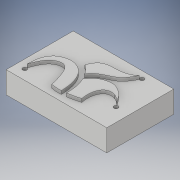
# Autodesk Inventor part: cimproj
Saved by Autodesk Inventor 2019 (Build 230136000, 136)
## iProperties
Created: 2021-02-26
Part Number: cimproj
Material: Generic
Document SubType Name: Modeling
Designer: Davron
Density: 1 g/cm^3
Appearance: Default
Author: Davron
Autodesk Inventor part; units mm, degrees
ref_plane "YZ Plane" through (0, 0, 0) normal (1, 0, 0) x (0, 1, 0)
ref_plane "XZ Plane" through (0, 0, 0) normal (0, 1, 0) x (-1, 0, 0)
ref_plane "XY Plane" through (0, 0, 0) normal (0, 0, 1) x (1, 0, 0)
sketch "Sketch1" plane through (0, 0, 0) normal (0, 1, 0) x (-1, 0, 0)
  line L0 (105.8864, -9.1713) -> (29.6864, -9.1713)
  line L1 (29.6864, -9.1713) -> (29.6864, -59.9713)
  line L2 (29.6864, -59.9713) -> (105.8864, -59.9713)
  line L3 (105.8864, -59.9713) -> (105.8864, -9.1713)
  point P0 (0, 0)
  dimension "d0" = 76.2
  dimension "d1" = 50.8
  constraints: 8 end point, 3 perpendicular, 1 horizontal
  measures "d0" distance of L0.start L0.end
  measures "d1" distance of L0.end L1.end
extrude "Extrusion1" add sketch "Sketch1" along normal blind 16.51
sketch "Sketch2" plane through (0, 16.51, 0) normal (0, 1, 0) x (1, 0, 0)
  line L0 (-99.1001, 18.3012) -> (-96.0417, 26.9953) construction
  line L1 (-96.0417, 26.9953) -> (-92.1887, 31.3423) construction
  line L2 (-92.1887, 31.3423) -> (-84.285, 34.3061) construction
  line L3 (-84.285, 34.3061) -> (-80.6296, 29.3664) construction
  line L4 (-80.6296, 29.3664) -> (-77.2705, 18.3012) construction
  line L5 (-77.2705, 18.3012) -> (-76.579, 14.4191) construction
  spline S0 degree 4 poles (-99.1001, 18.3012) (-96.0417, 26.9953) (-92.1887, 31.3423) (-84.285, 34.3061) (-80.6296, 29.3664) (-77.2705, 18.3012) (-76.579, 14.4191) knots 1 1 1 1 1 2 3 4 4 4 4 4
  line L6 (-99.1001, 18.3012) -> (-99.1001, 25.8499) construction
  line L7 (-99.1001, 25.8499) -> (-96.5674, 31.3423) construction
  line L8 (-96.5674, 31.3423) -> (-93.9607, 34.9573) construction
  line L9 (-93.9607, 34.9573) -> (-88.2369, 37.0386) construction
  line L10 (-88.2369, 37.0386) -> (-83.2313, 37.9368) construction
  line L11 (-83.2313, 37.9368) -> (-75.6293, 34.8836) construction
  line L12 (-75.6293, 34.8836) -> (-71.3593, 29.3664) construction
  line L13 (-71.3593, 29.3664) -> (-68.785, 20.2226) construction
  line L14 (-68.785, 20.2226) -> (-68.785, 13.8588) construction
  spline S1 degree 4 poles (-99.1001, 18.3012) (-99.1001, 25.8499) (-96.5674, 31.3423) (-93.9607, 34.9573) (-88.2369, 37.0386) (-83.2313, 37.9368) (-75.6293, 34.8836) (-71.3593, 29.3664) (-68.785, 20.2226) (-68.785, 13.8588) knots 1 1 1 1 1 2 3 4 5 6 7 7 7 7 7
  line L15 (-68.2598, 29.584) -> (-66.503, 25.2471) construction
  line L16 (-66.503, 25.2471) -> (-65.2915, 22.9111) construction
  line L17 (-65.2915, 22.9111) -> (-65.2915, 14.27) construction
  spline S2 degree 3 poles (-68.2598, 29.584) (-66.503, 25.2471) (-65.2915, 22.9111) (-65.2915, 14.27) knots 1 1 1 1 2 2 2 2
  spline S3 degree 2 poles (-70.7555, 33.4961) (-73.1331, 37.1458) (-76.6265, 39.605) knots 0 0 0 1 1 1
  line L18 (-76.6265, 39.605) -> (-71.5951, 54.9343) construction
  line L19 (-71.5951, 54.9343) -> (-60.3667, 43.5663) construction
  line L20 (-60.3667, 43.5663) -> (-49.0964, 53.1455) construction
  spline S4 degree 3 poles (-76.6265, 39.605) (-71.5951, 54.9343) (-60.3667, 43.5663) (-49.0964, 53.1455) knots 1 1 1 1 2 2 2 2
  line L21 (-65.2915, 14.27) -> (-59.8318, 14.9374) construction
  line L22 (-59.8318, 14.9374) -> (-55.9104, 16.3841) construction
  line L23 (-55.9104, 16.3841) -> (-55.7779, 16.3841) construction
  spline S5 degree 3 poles (-65.2915, 14.27) (-59.8318, 14.9374) (-55.9104, 16.3841) (-55.7779, 16.3841) knots 1 1 1 1 2 2 2 2
  line L24 (-57.1115, 22.9111) -> (-55.7779, 16.3841) construction
  spline S6 degree 4 poles (-45.7217, 31.3084) (-51.5634, 33.293) (-56.0482, 30.8036) (-57.1115, 22.9111) (-55.7779, 16.3841) knots 1.168057 1.168057 1.168057 1.168057 1.168057 2 2 2 2 2
  line L25 (-45.7217, 31.3084) -> (-51.5634, 33.293) construction
  line L26 (-51.5634, 33.293) -> (-56.0482, 30.8036) construction
  line L27 (-56.0482, 30.8036) -> (-57.1115, 22.9111) construction
  line L28 (-45.7217, 31.3084) -> (-43.5479, 30.466) construction
  line L29 (-43.5479, 30.466) -> (-40.4918, 27.639) construction
  spline S7 degree 2 poles (-45.7217, 31.3084) (-43.5479, 30.466) (-40.4918, 27.639) knots 1 1 1 2 2 2
  line L30 (-40.4918, 27.639) -> (-44.1138, 33.293) construction
  line L31 (-44.1138, 33.293) -> (-48.4479, 36.0572) construction
  line L32 (-48.4479, 36.0572) -> (-52.5651, 39.1817) construction
  line L33 (-52.5651, 39.1817) -> (-59.6522, 37.2966) construction
  line L34 (-59.6522, 37.2966) -> (-64.7462, 34.8183) construction
  line L35 (-64.7462, 34.8183) -> (-68.2598, 29.584) construction
  spline S8 degree 4 poles (-40.4918, 27.639) (-44.1138, 33.293) (-48.4479, 36.0572) (-52.5651, 39.1817) (-59.6522, 37.2966) (-64.7462, 34.8183) (-68.2598, 29.584) knots 1 1 1 1 1 2 3 4 4 4 4 4
  spline S9 degree 4 poles (-70.7555, 33.4961) (-66.7607, 40.5932) (-58.5336, 42.023) (-54.7819, 41.9147) (-49.0964, 53.1455) knots 0 0 0 0 0 1 1 1 1 1
  line L36 (-76.579, 14.4191) -> (-73.1385, 13.5025) construction
  line L37 (-73.1385, 13.5025) -> (-68.785, 13.8588) construction
  spline S10 degree 2 poles (-76.579, 14.4191) (-73.1385, 13.5025) (-68.785, 13.8588) knots 1 1 1 2 2 2
  point P0 (0, 0)
  point P1 (-73.4266, 36.8633)
  point P2 (-65.6468, 38.768)
  point P3 (-60.3715, 41.5372)
  point P4 (-55.5489, 44.3879)
  constraints: 3 vertical, 1 horizontal, 35 other
sketch "Sketch5" plane through (0, 16.51, 0) normal (0, 1, 0) x (1, 0, 0)
  circle A0 centre (-39.7111, 26.2451) radius 1.5875
  circle A1 centre (-99.3276, 16.7185) radius 1.5875
  circle A2 centre (-48.3267, 54.5366) radius 1.5875
  point P0 (0, 0)
  constraints: 3 centre point
extrude "Extrusion8" add sketch "Sketch2" along normal blind 2.54
extrude "Extrusion9" cut sketch "Sketch5" against normal blind 2.54
body "Solid1"
